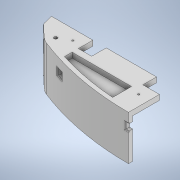
# Autodesk Inventor part: bumper_base_final _원본수정
Saved by Autodesk Inventor 2020 (Build 240168000, 168)
## iProperties
Created: 2022-06-30
Part Number: bumper_base_final _원본수정
Material: 일반
Document SubType Name: Modeling
Designer: samsung
Density: 1 g/cm^3
Appearance: 기본값
Author: samsung
Autodesk Inventor part; units mm, degrees
ref_plane "YZ Plane" through (0, 0, 0) normal (1, 0, 0) x (0, 1, 0)
ref_plane "XZ Plane" through (0, 0, 0) normal (0, 1, 0) x (-1, 0, 0)
ref_plane "XY Plane" through (0, 0, 0) normal (0, 0, 1) x (1, 0, 0)
sketch "스케치1" plane through (0, 0, 0) normal (0, 1, 0) x (-1, 0, 0)
  line L0 (-417.5, 136.0278) -> (167.5, 136.0278)
  arc A0 (126.8346, 86.699) -> (-406.6899, 73.6783) centre (-125, -531.4722) ccw
  line L1 (145.8326, 68.5278) -> (-85, 68.5278)
  line L2 (-165, 68.5278) -> (-393.8982, 68.5278)
  line L3 (-125, -531.4722) -> (-125, 1435.9267)
  circle A1 centre (-125, -531.4722) radius 1967.3989
  line L4 (-417.5444, 28.5399) -> (-406.6899, 73.6783)
  line L5 (-407.5098, 28.5399) -> (-398.3801, 66.5058)
  arc A2 (1441.9544, 38.2515) -> (-1691.7763, 38.7413) centre (-125, -531.4722) ccw
  line L6 (-371.3038, 78.1512) -> (-261.7019, 111.6599)
  line L7 (-261.7019, 111.6599) -> (11.7019, 111.6599)
  line L8 (-316.5029, 94.9056) -> (-320.1581, 106.8613)
  line L9 (-316.5029, 94.9056) -> (-397.3646, 1416.9826)
  line L10 (-316.5029, 94.9056) -> (-988.7616, 1236.1743)
  line L11 (-398.3844, 66.4971) -> (-125, -531.4722)
  line L12 (-407.5098, 28.5399) -> (-405.1717, 38.2627)
  line L13 (-405.1717, 38.2627) -> (-414.6578, 40.5439)
  line L14 (-405.1717, 38.2627) -> (-1671.8283, 684.2501)
  line L15 (-405.1717, 38.2627) -> (-2007.9181, 38.8589)
  line L16 (-405.1717, 38.2627) -> (-402.8337, 47.9856)
  line L17 (-402.8337, 47.9856) -> (-371.3038, 78.1512)
  line L18 (-387.0687, 63.0684) -> (-400.1089, 76.6983)
  line L19 (-387.0687, 63.0684) -> (-1557.9022, 816.656)
  line L20 (-387.0687, 63.0684) -> (-1051.9279, 1203.8846)
  line L21 (-125, -531.4722) -> (-261.7019, 111.6599)
  line L22 (-125, -531.4722) -> (11.7019, 111.6599)
  line L23 (-417.5444, 28.5399) -> (-407.5098, 28.5399)
  line L24 (-125, -531.4722) -> (-371.3038, 78.1512)
  line L25 (-125, -531.4722) -> (121.3038, 78.1512)
  line L26 (11.7019, 111.6599) -> (121.3038, 78.1512)
  line L27 (167.4556, 28.5399) -> (161.439, 53.6007)
  line L28 (121.3038, 78.1512) -> (152.8486, 47.9794)
  line L29 (157.5156, 28.5399) -> (167.4556, 28.5399)
  line L30 (-125, -531.4722) -> (148.2715, 66.1951)
  line L31 (-259.0118, 93.6599) -> (9.0118, 93.6599)
  line L32 (111.9521, 62.1879) -> (136.5817, 38.6304)
  line L33 (9.0118, 93.6599) -> (111.9521, 62.1879)
  line L34 (-361.9509, 62.1883) -> (-386.641, 38.5664)
  line L35 (-387.0049, 38.256) -> (-387.0101, 38.2515)
  line L36 (-388.9967, 28.5399) -> (-386.569, 38.6353)
  line L37 (-361.9509, 62.1883) -> (-259.0118, 93.6599)
  line L38 (-407.5098, 28.5399) -> (-388.9967, 28.5399)
  line L39 (136.5817, 38.6304) -> (139.0042, 28.5399)
  line L40 (157.5156, 28.5399) -> (139.0042, 28.5399)
  line L41 (-125, 111.6599) -> (-155, 111.6599)
  line L42 (-155, 111.6599) -> (-155, 93.6599)
  line L43 (-155, 93.6599) -> (-125, 93.6599)
  line L44 (-125, 93.6599) -> (-125, 111.6599)
  line L45 (152.8486, 47.9794) -> (145.0697, 46.1119)
  line L46 (145.0697, 46.1119) -> (148.5713, 31.5263)
  line L47 (148.5713, 31.5263) -> (156.3503, 33.3939)
  line L48 (137.0762, 63.0653) -> (129.8496, 69.9774)
  line L49 (129.8496, 69.9774) -> (124.32, 64.1961)
  line L50 (124.32, 64.1961) -> (138.7732, 50.372)
  line L51 (138.7732, 50.372) -> (144.3028, 56.1533)
  line L52 (66.5029, 94.9056) -> (56.9398, 97.8293)
  line L53 (56.9398, 97.8293) -> (54.6009, 90.1788)
  line L54 (54.6009, 90.1788) -> (73.727, 84.3314)
  line L55 (73.727, 84.3314) -> (76.0659, 91.9818)
  line L56 (76.0659, 91.9818) -> (66.5029, 94.9056)
  line L57 (-125, 111.6599) -> (-135, 111.6599)
  line L58 (-135, 111.6599) -> (-135, 103.6599)
  line L59 (-135, 103.6599) -> (-115, 103.6599)
  line L60 (-115, 103.6599) -> (-115, 111.6599)
  line L61 (-115, 111.6599) -> (-125, 111.6599)
  line L62 (161.439, 53.6007) -> (126.8346, 86.699)
  arc A3 (121.3038, 78.1512) -> (-398.3844, 66.4971) centre (-125, -531.4722) ccw
  line L63 (157.5156, 28.5399) -> (152.8486, 47.9794)
  line L64 (139.0042, 28.5399) -> (-125, 28.5399)
  line L65 (-85, 124.81) -> (-85, 0)
  line L66 (-125, 0) -> (-125, 61.5)
  line L67 (-125, 61.5) -> (-85, 61.5)
  line L68 (-85, 61.5) -> (-75, 61.5)
  line L69 (-75, 61.5) -> (-75, 124.1239)
  line L70 (91.215, 68.5278) -> (91.215, 89.4604)
  line L71 (-125, 28.5399) -> (-125, 78.5399)
  line L72 (-125, 78.5399) -> (91.215, 78.5399)
  line L73 (-75, 61.5) -> (-75, 28.5399)
  line L74 (68, 97.0636) -> (68, 28.5399)
  point P0 (0, 0)
  point P1 (0, 0)
  point P2 (143.8982, 61.5)
  point P3 (-393.8982, 61.5)
  point P4 (-417.5, 21.5)
  point P5 (-165, 0)
  point P6 (-85, 0)
  point P7 (-85, 12.4229)
  point P8 (167.5, 12.4229)
  point P9 (-393.8982, -388.5)
  point P10 (-165, -388.5)
  point P11 (167.5, -327)
  point P12 (-417.5, -327)
  point P13 (-85, -388.5)
  point P14 (143.8982, -388.5)
  point P15 (162, 21.5)
  point P16 (162, 12.4229)
  point P17 (167.5, 21.5)
  point P18 (-125, 0)
  point P19 (-125, 136.0278)
  point P20 (-125, 136.0278)
  point P21 (-125, 93.6599)
  point P22 (-155, 111.6599)
  point P23 (-398.3829, 66.4939)
  point P24 (128.4632, 68.5278)
  point P25 (131.3651, 68.5278)
  point P26 (-125, 103.6599)
  point P27 (143.8695, 56.5677)
  point P28 (143.1097, 54.9059)
  point P29 (-125, 126.0278)
  point P30 (-85, 28.5399)
  point P31 (-75, 68.5278)
  point P32 (-75, 78.5399)
  point P33 (58.467, 78.5399)
  point P34 (68, 75.6254)
  dimension "d13" = 667.5
  dimension "d15" = 585
  dimension "d25" = 1299.8989
  dimension "d39" = 999.8126
  dimension "d45" = 13.5
  dimension "d46" = 13.5
  dimension "d50" = 10
  dimension "d51" = 13.5
  dimension "d52" = 13.5
  dimension "d53" = 10
  dimension "d54" = 13.5
  dimension "d55" = 13.5
  dimension "d56" = 12
  dimension "d57" = 12
  dimension "d60" = 10
  dimension "d72" = 10
  dimension "d81" = 18
  dimension "d83" = 18
  dimension "d84" = 18
  dimension "d85" = 18
  dimension "d126" = 30
  dimension "d163" = 8
  dimension "d164" = 15
  dimension "d165" = 10
  dimension "d166" = 8
  dimension "d167" = 20
  dimension "d168" = 10
  dimension "d169" = 8
  dimension "d170" = 20
  dimension "d171" = 10
  dimension "d172" = 8
  dimension "d173" = 20
  dimension "d182" = 10
  dimension "d190" = 61.5
  dimension "d191" = 10
  dimension "d203" = 50
  dimension "d256" = 143
  constraints: 150 end point, 28 point on line, 23 perpendicular, 10 parallel, 7 horizontal, 7 point on circle, 6 midpoint, 2 centre point, 2 collinear, 1 coincident, 1 tangent, 1 vertical, 23 other
  measures "d13" radius of A0
  measures "d15" distance of L27.start L4.start
  measures "d39" radial gap between concentric circles of A0 A2
  measures "d45" angle of L8 L9
  measures "d46" angle of L10 L8
  measures "d50" distance of L5.start L12.end
  measures "d51" angle of L14 L13
  measures "d52" angle of L15 L13
  measures "d53" distance of L12.end L16.end
  measures "d54" angle of L18 L20
  measures "d55" angle of L18 L19
  measures "d56" angle of L3 L21
  measures "d57" angle of L22 L3
  measures "d60" angle of L24 L21
  measures "d72" angle of L25 L22
  measures "d81" distance between parallel lines of L7 L31
  measures "d83" distance between parallel lines of L28 L32
  measures "d84" distance between parallel lines of L17 L34
  measures "d85" distance between parallel lines of L12 L36
  measures "d126" distance of L42.end L43.end
  measures "d163" distance of L28.end L45.end
  measures "d164" distance of L45.end L46.end
  measures "d165" distance of L48.start L48.end
  measures "d166" distance of L48.end L49.end
  measures "d167" distance of L49.end L50.end
  measures "d168" distance of L52.start L52.end
  measures "d169" distance of L52.end L53.end
  measures "d170" distance of L53.end L54.end
  measures "d171" distance of L41.start L57.end
  measures "d172" distance of L57.end L58.end
  measures "d173" distance of L58.end L59.end
  measures "d182" distance between parallel lines of L62 L28
  measures "d190" distance of L66.start L66.end
  measures "d191" distance of L67.end L68.end
  measures "d203" distance of L64.end L71.end
  measures "d256" distance between parallel lines of L74 L73
extrude "돌출11" add sketch "스케치1" against normal blind 90 contours A0 L62 L1 L28 A3 L3 | L62 L30 L28 L1 | L62 L27 L29 L63 L28 L30
ref_plane "작업 평면1" through (-148.5713, -30, 31.5263) normal (-0.9723699, 0, 0.2334454) x (0.2334454, 0, 0.9723699)
sketch "스케치15" plane through (-148.5713, -30, 31.5263) normal (-0.9723699, 0, 0.2334454) x (0.2334454, 0, 0.9723699)
  line L0 (0, 30) -> (15, 30)
  line L1 (0, 30) -> (0, 0)
  line L2 (15, 0) -> (0, 0)
  line L3 (15, 30) -> (15, 0)
  line L4 (11.5, 7.5) -> (3.5, 7.5)
  line L5 (3.5, 7.5) -> (3.5, 22.5)
  line L6 (3.5, 22.5) -> (11.5, 22.5)
  line L7 (11.5, 22.5) -> (11.5, 7.5)
  line L8 (11.5, 7.5) -> (3.5, 22.5) construction
  line L9 (3.5, 7.5) -> (11.5, 22.5) construction
  point P0 (7.5, 15)
  point P1 (7.5, 15)
  point P2 (0, 15)
  dimension "d174" = 8
  dimension "d175" = 15
  constraints: 20 end point, 4 midpoint, 2 parallel, 1 horizontal, 1 horizontal alignment, 1 perpendicular, 4 other
  measures "d174" distance of L5.end L6.end
  measures "d175" distance of L4.end L5.end
extrude "돌출13" cut sketch "스케치15" along normal blind 30 contours L4 L5 L6 L7
ref_plane "작업 평면2" through (-138.7732, -30, 50.372) normal (-0.6912048, 0, 0.7226589) x (0.7226589, 0, 0.6912048)
sketch "스케치16" plane through (-138.7732, -30, 50.372) normal (-0.6912048, 0, 0.7226589) x (0.7226589, 0, 0.6912048)
  line L0 (0, 30) -> (20, 30)
  line L1 (0, 30) -> (0, 0)
  line L2 (20, 0) -> (0, 0)
  line L3 (20, 30) -> (20, 0)
  line L4 (2.5, 22.5) -> (17.5, 22.5)
  line L5 (17.5, 22.5) -> (17.5, 7.5)
  line L6 (17.5, 7.5) -> (2.5, 7.5)
  line L7 (2.5, 7.5) -> (2.5, 22.5)
  line L8 (2.5, 22.5) -> (17.5, 7.5) construction
  line L9 (17.5, 22.5) -> (2.5, 7.5) construction
  point P0 (10, 15)
  point P1 (10, 15)
  point P2 (10, 0)
  dimension "d230" = 15
  dimension "d231" = 15
  constraints: 20 end point, 3 midpoint, 2 parallel, 1 horizontal, 1 perpendicular, 1 vertical alignment
  measures "d230" distance of L5.end L6.end
  measures "d231" distance of L4.end L5.end
extrude "돌출14" cut sketch "스케치16" along normal blind 30 contours L4 L5 L6 L7
ref_plane "작업 평면3" through (-73.727, -30, 84.3314) normal (-0.2923717, 0, 0.9563048) x (0.9563048, 0, 0.2923717)
sketch "스케치17" plane through (-73.727, -30, 84.3314) normal (-0.2923717, 0, 0.9563048) x (0.9563048, 0, 0.2923717)
  line L0 (0, 30) -> (20, 30)
  line L1 (0, 30) -> (0, 0)
  line L2 (20, 0) -> (0, 0)
  line L3 (20, 30) -> (20, 0)
  line L4 (17.5, 22.5) -> (2.5, 22.5)
  line L5 (2.5, 22.5) -> (2.5, 7.5)
  line L6 (2.5, 7.5) -> (17.5, 7.5)
  line L7 (17.5, 7.5) -> (17.5, 22.5)
  line L8 (17.5, 22.5) -> (2.5, 7.5) construction
  line L9 (2.5, 22.5) -> (17.5, 7.5) construction
  point P0 (10, 15)
  dimension "d228" = 15
  dimension "d229" = 15
  constraints: 20 end point, 2 midpoint, 2 parallel, 1 horizontal, 1 perpendicular
  measures "d228" distance of L6.end L5.end
  measures "d229" distance of L5.end L4.end
extrude "돌출15" cut sketch "스케치17" along normal blind 30 contours L7 L6 L5 L4
ref_plane "작업 평면4" through (115, 0, 103.6599) normal (0, 0, 1) x (1, 0, 0)
sketch "스케치18" plane through (115, 0, 103.6599) normal (0, 0, 1) x (1, 0, 0)
  line L0 (0, 0) -> (0, -30)
  line L1 (10, -30) -> (0, -30)
  line L2 (2.5, -7.5) -> (17.5, -7.5)
  line L3 (17.5, -7.5) -> (17.5, -22.5)
  line L4 (17.5, -22.5) -> (2.5, -22.5)
  line L5 (2.5, -22.5) -> (2.5, -7.5)
  line L6 (2.5, -7.5) -> (17.5, -22.5) construction
  line L7 (17.5, -7.5) -> (2.5, -22.5) construction
  line L8 (10, 0) -> (10, -30)
  line L9 (0, 0) -> (10, 0)
  point P0 (10, -15)
  point P1 (10, -15)
  point P2 (10, -22.5)
  point P3 (10, -7.5)
  point P4 (10, -15)
  dimension "d225" = 10
  dimension "d226" = 15
  dimension "d227" = 15
  constraints: 20 end point, 4 midpoint, 2 horizontal, 2 parallel, 1 perpendicular, 1 vertical, 1 vertical alignment, 3 other
  measures "d225" distance of L0.start L8.start
  measures "d226" distance of L3.end L4.end
  measures "d227" distance of L2.end L3.end
extrude "돌출16" cut sketch "스케치18" along normal blind 50 contours L8 L4 L5 L2
extrude "돌출17" add sketch "스케치1" along normal blind 17 contours A0 L62 L1 L28 A3 L3 | A3 L65 L7 L3 | L62 L30 L28 L1 | L7 L60 L59 L3 | A3 L69 L7 L65 | L28 L30 L51 L50 L49 L1 | L1 L49 L28 | L62 L27 L29 L63 L28 L30 | L59 L60 L7 L65 L31 L3 | L7 L69 L31 L65 | L49 L50 L51 L30 L32 L25 L1 | L1 L25 L28 L49 | L28 L51 L30 | L31 L65 L72 L3 | L31 L69 L72 L65 | L25 L32 L33 L1 | L1 L70 L26 L25 | L26 L70 A3 | L28 L45 L46 L47 L63 L40 L39 L32 L30 L51 | L72 L65 L67 L3 | A3 L70 L26 L74 | L72 L69 L1 L65 | L64 L74 L1 L33 L32 L25 | L25 L32 L30 L64 | L30 L32 L39 L64 | L1 L74 L33 | L33 L74 L72 L70 | L70 L72 L74 L54 L55 L26 | L63 L47 L46 L45 | L26 L55 L54 L74 | L1 L69 L68 L65
sketch "스케치19" plane through (0, 17, 0) normal (0, 1, 0) x (1, 0, 0)
  line L0 (-161.439, -53.6007) -> (-126.8346, -86.699) projected
  arc A0 (-126.8346, -86.699) -> (125, -136.0278) centre (125, 531.4722) ccw projected
  line L1 (125, -136.0278) -> (125, -61.5) projected
  line L2 (125, -61.5) -> (75, -61.5) projected
  line L3 (-68, -28.5399) -> (-167.4556, -28.5399) projected
  line L4 (-167.4556, -28.5399) -> (-161.439, -53.6007) projected
  line L5 (75, -61.5) -> (75, -124.1239) projected
  arc A1 (-68, -97.0636) -> (75, -124.1239) centre (125, 531.4722) ccw projected
  line L6 (-9.0118, -93.6599) -> (-111.9521, -62.1879) projected
  line L7 (-11.7019, -111.6599) -> (-121.3038, -78.1512) projected
  line L8 (-111.9521, -62.1879) -> (-136.5817, -38.6304) projected
  line L9 (-136.5817, -38.6304) -> (-139.0042, -28.5399) projected
  line L10 (-121.3038, -78.1512) -> (-152.8486, -47.9794) projected
  line L11 (-152.8486, -47.9794) -> (-157.5156, -28.5399) projected
  line L12 (-157.5156, -28.5399) -> (-139.0042, -28.5399) projected
  circle A2 centre (-117.5156, -68.5399) radius 3.6
  line L13 (-119.5941, -72.1399) -> (-121.6726, -68.5399)
  line L14 (-121.6726, -68.5399) -> (-119.5941, -64.9399)
  line L15 (-119.5941, -64.9399) -> (-115.4372, -64.9399)
  line L16 (-115.4372, -64.9399) -> (-113.3587, -68.5399)
  line L17 (-113.3587, -68.5399) -> (-115.4372, -72.1399)
  line L18 (-115.4372, -72.1399) -> (-119.5941, -72.1399)
  line L19 (-68, -97.0636) -> (-68, -28.5399) projected
  point P0 (0, 0)
  point P1 (-91.215, -68.5278)
  point P2 (-117.5156, -72.1399)
  dimension "d196" = 7.2
  dimension "d194" = 40
  dimension "d195" = 40
  constraints: 12 end point, 2 coincident, 1 midpoint, 1 vertical alignment, 15 other
  measures "d194" distance from line of L3 point (-117.516, -68.54)
  measures "d195" horizontal distance of point (-117.516, -68.54) L11.end
extrude "돌출18" cut sketch "스케치19" against normal blind 10 contours A2 | A2 L16 L17 | A2 L15 L16 | L17 L18 A2 | A2 L14 L15 | L18 L13 A2 | A2 L13 L14
sketch "스케치21" plane through (0, 7, 0) normal (0, 1, 0) x (1, 0, 0)
  line L0 (-115.4372, -64.9399) -> (-113.3587, -68.5399) projected
  line L1 (-119.5941, -64.9399) -> (-115.4372, -64.9399) projected
  line L2 (-121.6726, -68.5399) -> (-119.5941, -64.9399) projected
  line L3 (-119.5941, -72.1399) -> (-121.6726, -68.5399) projected
  line L4 (-115.4372, -72.1399) -> (-119.5941, -72.1399) projected
  line L5 (-113.3587, -68.5399) -> (-115.4372, -72.1399) projected
  point P0 (0, 0)
  point P1 (-117.5156, -68.5399)
hole "구멍3" at (-117.5156, 7, 68.5399) direction (0, -1, 0) diameter 4.2 end through all
sketch "스케치22" plane through (0, 0, 0) normal (0, -1, 0) x (1, 0, 0)
  line L0 (75, 61.5) -> (75, 124.1239) projected
  line L1 (125, 61.5) -> (75, 61.5) projected
  line L2 (-68, 28.5399) -> (-157.5156, 28.5399) projected
  circle A0 centre (100, 86.5) radius 3.6
  circle A1 centre (-91.215, 53.5399) radius 3.6
  line L3 (97.9215, 82.9) -> (95.8431, 86.5)
  line L4 (95.8431, 86.5) -> (97.9215, 90.1)
  line L5 (97.9215, 90.1) -> (102.0785, 90.1)
  line L6 (102.0785, 90.1) -> (104.1569, 86.5)
  line L7 (104.1569, 86.5) -> (102.0785, 82.9)
  line L8 (102.0785, 82.9) -> (97.9215, 82.9)
  line L9 (-93.2935, 49.9399) -> (-95.372, 53.5399)
  line L10 (-95.372, 53.5399) -> (-93.2935, 57.1399)
  line L11 (-93.2935, 57.1399) -> (-89.1366, 57.1399)
  line L12 (-89.1366, 57.1399) -> (-87.0581, 53.5399)
  line L13 (-87.0581, 53.5399) -> (-89.1366, 49.9399)
  line L14 (-89.1366, 49.9399) -> (-93.2935, 49.9399)
  point P0 (0, 0)
  point P1 (100, 82.9)
  point P2 (-91.215, 49.9399)
  dimension "d214" = 7.2
  dimension "d215" = 7.2
  dimension "d211" = 25
  dimension "d212" = 25
  dimension "d213" = 25
  constraints: 24 end point, 4 coincident, 2 midpoint, 2 vertical alignment, 30 other
  measures "d211" distance from line of L0 point (100, 86.5)
  measures "d212" distance from line of L1 point (100, 86.5)
  measures "d213" distance from line of L2 point (-91.215, 53.54)
extrude "돌출19" cut sketch "스케치22" against normal blind 10
sketch "스케치23" plane through (0, 10, 0) normal (0, -1, 0) x (1, 0, 0)
  line L0 (97.9215, 90.1) -> (102.0785, 90.1) projected
  line L1 (95.8431, 86.5) -> (97.9215, 90.1) projected
  line L2 (97.9215, 82.9) -> (95.8431, 86.5) projected
  line L3 (102.0785, 82.9) -> (97.9215, 82.9) projected
  line L4 (104.1569, 86.5) -> (102.0785, 82.9) projected
  line L5 (102.0785, 90.1) -> (104.1569, 86.5) projected
  line L6 (-89.1366, 57.1399) -> (-87.0581, 53.5399) projected
  line L7 (-93.2935, 57.1399) -> (-89.1366, 57.1399) projected
  line L8 (-95.372, 53.5399) -> (-93.2935, 57.1399) projected
  line L9 (-93.2935, 49.9399) -> (-95.372, 53.5399) projected
  line L10 (-89.1366, 49.9399) -> (-93.2935, 49.9399) projected
  line L11 (-87.0581, 53.5399) -> (-89.1366, 49.9399) projected
  point P0 (0, 0)
  point P1 (100, 86.5)
  point P2 (-91.215, 53.5399)
hole "구멍4" at (100, 10, 86.5) at (-91.215, 10, 53.5399) direction (0, 1, 0) diameter 4.2 end through all
sketch "스케치24" plane through (-167.4556, -90, 28.5399) normal (-0.9723699, 0, 0.2334454) x (0.2334454, 0, 0.9723699)
  line L0 (18.8123, 67.5) -> (10.8123, 67.5) projected
  line L1 (10.8123, 67.5) -> (10.8123, 82.5) projected
  line L2 (10.8123, 82.5) -> (18.8123, 82.5) projected
  line L3 (18.8123, 82.5) -> (18.8123, 67.5) projected
  line L4 (7.3123, 65) -> (22.3123, 65)
  line L5 (22.3123, 65) -> (22.3123, 85)
  line L6 (22.3123, 85) -> (7.3123, 85)
  line L7 (7.3123, 85) -> (7.3123, 65)
  line L8 (7.3123, 65) -> (22.3123, 85) construction
  line L9 (22.3123, 65) -> (7.3123, 85) construction
  point P0 (14.8123, 75)
  point P1 (14.8123, 75)
  point P2 (14.8123, 82.5)
  dimension "d232" = 15
  dimension "d233" = 20
  constraints: 12 end point, 4 midpoint, 2 parallel, 1 horizontal, 1 perpendicular, 1 vertical alignment
  measures "d232" distance of L6.end L5.end
  measures "d233" distance of L5.end L4.end
extrude "돌출20" cut sketch "스케치24" against normal blind 2 contours L0 L1 L2 L3 | L7 L6 L5 L4
sketch "스케치25" plane through (-161.439, -90, 53.6007) normal (-0.6912048, 0, 0.7226589) x (0.7226589, 0, 0.6912048)
  line L0 (16.648, 82.5) -> (31.648, 82.5) projected
  line L1 (16.648, 67.5) -> (16.648, 82.5) projected
  line L2 (31.648, 67.5) -> (16.648, 67.5) projected
  line L3 (31.648, 82.5) -> (31.648, 67.5) projected
  line L4 (14.148, 85) -> (34.148, 85)
  line L5 (34.148, 85) -> (34.148, 65)
  line L6 (34.148, 65) -> (14.148, 65)
  line L7 (14.148, 65) -> (14.148, 85)
  line L8 (14.148, 85) -> (34.148, 65) construction
  line L9 (34.148, 85) -> (14.148, 65) construction
  point P0 (24.148, 75)
  dimension "d236" = 20
  dimension "d237" = 20
  constraints: 12 end point, 2 midpoint, 2 parallel, 1 horizontal, 1 perpendicular
  measures "d236" distance of L5.end L6.end
  measures "d237" distance of L4.end L5.end
extrude "돌출21" cut sketch "스케치25" against normal blind 2 contours L0 L3 L2 L1 | L4 L5 L6 L7
ref_plane "작업 평면5" through (-77.3181, -7.5, 104.6282) normal (0.2923717, 0, -0.9563048) x (0.9563048, 0, 0.2923717)
sketch "스케치26" plane through (-77.3181, -7.5, 104.6282) normal (0.2923717, 0, -0.9563048) x (0.9563048, 0, 0.2923717)
  line L0 (0, 15) -> (0, 0) projected
  line L1 (0, 0) -> (15, 0) projected
  line L2 (15, 0) -> (15, 15) projected
  line L3 (15, 15) -> (0, 15) projected
  line L4 (-2.5, -2.5) -> (17.5, -2.5)
  line L5 (17.5, -2.5) -> (17.5, 17.5)
  line L6 (17.5, 17.5) -> (-2.5, 17.5)
  line L7 (-2.5, 17.5) -> (-2.5, -2.5)
  line L8 (-2.5, -2.5) -> (17.5, 17.5) construction
  line L9 (17.5, -2.5) -> (-2.5, 17.5) construction
  point P0 (43.3493, -7.5)
  point P1 (7.5, 7.5)
  dimension "d240" = 20
  dimension "d241" = 20
  constraints: 12 end point, 2 midpoint, 2 parallel, 1 horizontal, 1 perpendicular
  measures "d240" distance of L6.end L5.end
  measures "d241" distance of L5.end L4.end
extrude "돌출22" cut sketch "스케치26" along normal mid plane 4 contours L3 L2 L1 L0 | L7 L6 L5 L4
ref_plane "작업 평면6" through (125, -7.5, 136.0278) normal (-0.0056181, 0, 0.9999842) x (-0.9999842, 0, -0.0056181)
sketch "스케치27" plane through (125, -7.5, 136.0278) normal (-0.0056181, 0, 0.9999842) x (-0.9999842, 0, -0.0056181)
  line L0 (0, 0) -> (7.5001, 0) projected
  line L1 (7.5001, 15) -> (7.5001, 0) projected
  line L2 (7.5001, 15) -> (0, 15) projected
  line L3 (0, 15) -> (0, 82.5) projected
  line L4 (10, -2.5) -> (0, -2.5)
  line L5 (0, 17.5) -> (10, 17.5)
  line L6 (10, 17.5) -> (10, -2.5)
  line L7 (0, -2.5) -> (0, 17.5)
  line L8 (0, 0) -> (0, -24.5) projected
  point P0 (125.7622, -7.5)
  point P1 (0, 7.5)
  point P2 (0, 7.5)
  dimension "d246" = 20
  dimension "d247" = 10
  constraints: 8 end point, 2 point on line, 1 coincident, 1 collinear, 1 horizontal, 1 midpoint, 1 parallel
  measures "d246" distance of L4.end L5.start
  measures "d247" distance of L4.start L4.end
extrude "돌출23" cut sketch "스케치27" along normal mid plane 4
fillet "모깎기4" radius 10 1 edges at (-161.439, -36.5, 53.6007)
fillet "모깎기5" radius 50 1 edges at (-126.8346, -36.5, 86.699)
sketch "스케치29" plane through (0, 17, 0) normal (0, 1, 0) x (1, 0, 0)
  circle A0 centre (100, -86.5) radius 2.1 projected
  circle A1 centre (-91.215, -53.5399) radius 2.1 projected
  line L0 (-115.4372, -72.1399) -> (-119.5941, -72.1399) projected
  line L1 (-119.5941, -72.1399) -> (-121.6726, -68.5399) projected
  line L2 (-121.6726, -68.5399) -> (-119.5941, -64.9399) projected
  line L3 (-119.5941, -64.9399) -> (-115.4372, -64.9399) projected
  line L4 (-115.4372, -64.9399) -> (-113.3587, -68.5399) projected
  line L5 (-113.3587, -68.5399) -> (-115.4372, -72.1399) projected
  arc A2 (-133.8532, -79.9858) -> (-117.4544, -90.4379) centre (-99.293, -43.8529) ccw projected
  arc A3 (-117.4544, -90.4379) -> (125, -136.0278) centre (125, 531.4722) ccw projected
  line L6 (125, -136.0278) -> (125, -61.5) projected
  line L7 (125, -61.5) -> (75, -61.5) projected
  line L8 (75, -61.5) -> (75, -124.1239) projected
  arc A4 (-68, -97.0636) -> (75, -124.1239) centre (125, 531.4722) ccw projected
  line L9 (-68, -97.0636) -> (-68, -28.5399) projected
  line L10 (-68, -28.5399) -> (-167.4556, -28.5399) projected
  line L11 (-167.4556, -28.5399) -> (-162.1255, -50.7412) projected
  arc A5 (-162.1255, -50.7412) -> (-159.3139, -55.6334) centre (-152.4018, -48.4068) ccw projected
  line L12 (-159.3139, -55.6334) -> (-133.8532, -79.9858) projected
  line L13 (75, -61.5) -> (75, -124.1239) projected
  line L14 (-68, -28.5399) -> (75, -28.5399)
  line L15 (75, -28.5399) -> (75, -78.5399)
  line L16 (75, -78.5399) -> (-68, -78.5399)
  line L17 (-68, -78.5399) -> (-68, -28.5399)
  line L18 (75, -61.5) -> (-36, -61.5)
  line L19 (-68, -97.0636) -> (-68, -28.5399) projected
  line L20 (75, -38.5399) -> (-68, -38.5399)
  line L21 (-36, -63.5399) -> (-68, -63.5399)
  line L22 (125, -61.5) -> (75, -61.5) projected
  line L23 (75, -28.5399) -> (85, -28.5399)
  line L24 (85, -28.5399) -> (85, -61.5)
  line L25 (85, -61.5) -> (75, -61.5)
  line L26 (75, -61.5) -> (75, -28.5399)
  line L27 (-36, -78.5399) -> (-36, -28.5399)
  point P0 (0, 0)
  point P1 (-68, -78.5399)
  point P2 (-68, -61.5)
  dimension "d257" = 50
  dimension "d258" = 10
  dimension "d264" = 35
  constraints: 24 end point, 7 point on line, 4 parallel, 4 perpendicular, 3 horizontal, 1 vertical
  measures "d257" distance between parallel lines of L14 L16
  measures "d258" distance between parallel lines of L14 L20
  measures "d264" distance between parallel lines of L14 L21
extrude "돌출24" add sketch "스케치29" against normal blind 12.3 contours L7 L15 L23 L24 | L18 L27 L20 L15 | L8 L16 L27 L18 | L14 L15 L20 L27 | L21 L27 L16 L9
sketch "스케치30" plane through (0, 0, 0) normal (0, -1, 0) x (1, 0, 0)
  line L0 (95.8431, 86.5) -> (97.9215, 90.1) projected
  line L1 (97.9215, 90.1) -> (102.0785, 90.1) projected
  line L2 (102.0785, 90.1) -> (104.1569, 86.5) projected
  line L3 (104.1569, 86.5) -> (102.0785, 82.9) projected
  line L4 (102.0785, 82.9) -> (97.9215, 82.9) projected
  line L5 (97.9215, 82.9) -> (95.8431, 86.5) projected
  arc A0 (125, 126.0278) -> (75, 124.1239) centre (125, -531.4722) ccw projected
  line L6 (75, 61.5) -> (75, 124.1239) projected
  line L7 (125, 61.5) -> (75, 61.5) projected
  line L8 (125, 126.0278) -> (125, 61.5) projected
  line L9 (-89.1366, 49.9399) -> (-93.2935, 49.9399) projected
  line L10 (-93.2935, 49.9399) -> (-95.372, 53.5399) projected
  line L11 (-95.372, 53.5399) -> (-93.2935, 57.1399) projected
  line L12 (-93.2935, 57.1399) -> (-89.1366, 57.1399) projected
  line L13 (-89.1366, 57.1399) -> (-87.0581, 53.5399) projected
  line L14 (-87.0581, 53.5399) -> (-89.1366, 49.9399) projected
  circle A1 centre (-117.5156, 68.5399) radius 2.1 projected
  line L15 (-152.8486, 47.9794) -> (-157.5156, 28.5399) projected
  line L16 (-68, 28.5399) -> (-157.5156, 28.5399) projected
  line L17 (-68, 97.0636) -> (-68, 28.5399) projected
  arc A2 (-68, 97.0636) -> (-121.3038, 78.1512) centre (125, -531.4722) ccw projected
  line L18 (-121.3038, 78.1512) -> (-152.8486, 47.9794) projected
  point P0 (0, 0)
extrude "돌출25" cut sketch "스케치30" against normal up to surface (4.7 mm away)
sketch "스케치31" plane through (0, 4.7, 0) normal (0, -1, 0) x (1, 0, 0)
  line L0 (-89.1366, 49.9399) -> (-87.0581, 53.5399) projected
  line L1 (-93.2935, 49.9399) -> (-89.1366, 49.9399) projected
  line L2 (-95.372, 53.5399) -> (-93.2935, 49.9399) projected
  line L3 (-93.2935, 57.1399) -> (-95.372, 53.5399) projected
  line L4 (-89.1366, 57.1399) -> (-93.2935, 57.1399) projected
  line L5 (-87.0581, 53.5399) -> (-89.1366, 57.1399) projected
  circle A0 centre (-117.5156, 68.5399) radius 2.1 projected
  line L6 (102.0785, 90.1) -> (97.9215, 90.1) projected
  line L7 (104.1569, 86.5) -> (102.0785, 90.1) projected
  line L8 (102.0785, 82.9) -> (104.1569, 86.5) projected
  line L9 (97.9215, 82.9) -> (102.0785, 82.9) projected
  line L10 (95.8431, 86.5) -> (97.9215, 82.9) projected
  line L11 (97.9215, 90.1) -> (95.8431, 86.5) projected
  line L12 (85, 28.5399) -> (85, 61.5) projected
  line L13 (125, 61.5) -> (85, 61.5) projected
  line L14 (125, 126.0278) -> (125, 61.5) projected
  arc A1 (125, 126.0278) -> (75, 124.1239) centre (125, -531.4722) ccw projected
  line L15 (75, 78.5399) -> (75, 124.1239) projected
  line L16 (75, 78.5399) -> (-68, 78.5399) projected
  line L17 (-68, 97.0636) -> (-68, 78.5399) projected
  arc A2 (-68, 97.0636) -> (-121.3038, 78.1512) centre (125, -531.4722) ccw projected
  line L18 (-152.8486, 47.9794) -> (-121.3038, 78.1512) projected
  line L19 (-157.5156, 28.5399) -> (-152.8486, 47.9794) projected
  line L20 (-68, 28.5399) -> (-157.5156, 28.5399) projected
  line L21 (-68, 28.5399) -> (-157.5156, 28.5399) projected
  arc A3 (125, 126.0278) -> (-121.3038, 78.1512) centre (125, -531.4722) ccw projected
  line L22 (125, 126.0278) -> (125, 61.5) projected
  line L23 (85, 42.5399) -> (-36, 42.5399)
  line L24 (-68, 42.5399) -> (-154.1545, 42.5399)
  line L25 (-68, 63.5399) -> (-68, 28.5399) projected
  line L26 (-36, 28.5399) -> (85, 28.5399) projected
  line L27 (-68, 63.5399) -> (-36, 63.5399) projected
  line L28 (-36, 63.5399) -> (-36, 28.5399) projected
  point P0 (0, 0)
  point P1 (75, 28.5399)
  constraints: 4 end point, 2 horizontal, 2 point on line
extrude "돌출26" add sketch "스케치31" along normal blind 4.7 contours L15 L16 L17 A3
equation "\"d46\" = d45"
equation "\"d57\" = d56"
equation "\"d72\" = d60"
equation "\"d61\" = d60"
